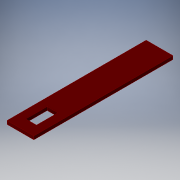
# Autodesk Inventor part: Brazo_Superior
Saved by Autodesk Inventor 2019 (Build 230136000, 136)
## iProperties
Created: 2020-02-09
Part Number: Brazo_Superior
Material: Generic
Document SubType Name: Modeling
Designer: Omar
Density: 1 g/cm^3
Appearance: Default
Author: Omar
Autodesk Inventor part; units mm, degrees
ref_plane "YZ Plane" through (0, 0, 0) normal (1, 0, 0) x (0, 1, 0)
ref_plane "XZ Plane" through (0, 0, 0) normal (0, 1, 0) x (-1, 0, 0)
ref_plane "XY Plane" through (0, 0, 0) normal (0, 0, 1) x (1, 0, 0)
sketch "Sketch1" plane through (0, 0, 0) normal (0, 1, 0) x (-1, 0, 0)
  line L0 (-7.5, -95.91) -> (-7.5, -99.09)
  line L1 (1.59, -90) -> (-1.59, -90)
  line L2 (-1.59, -90) -> (-1.59, -105)
  line L3 (-1.59, -105) -> (1.59, -105)
  line L4 (1.59, -105) -> (1.59, -90)
  line L5 (-1.59, -90) -> (1.59, -105) construction
  line L6 (7.5, -95.91) -> (-7.5, -95.91)
  line L7 (-7.5, -99.09) -> (7.5, -99.09)
  line L8 (7.5, -99.09) -> (7.5, -95.91)
  line L9 (1.59, -90) -> (-1.59, -105) construction
  line L10 (-5, 10) -> (5, 10)
  line L11 (5, 10) -> (5, -10)
  line L12 (5, -10) -> (-5, -10)
  line L13 (-5, -10) -> (-5, 10)
  line L14 (-5, 10) -> (5, -10) construction
  line L15 (5, 10) -> (-5, -10) construction
  line L16 (12.5, 20) -> (-12.5, 20)
  line L17 (-12.5, 20) -> (-12.5, -110)
  line L18 (-12.5, -110) -> (12.5, -110)
  line L19 (12.5, -110) -> (12.5, 20)
  point P0 (0, 0)
  point P1 (0, 0)
  point P2 (0, -97.5)
  point P3 (0, 0)
  dimension "d16" = 15
  dimension "d18" = 3.18
  dimension "d19" = 15
  dimension "d20" = 7.5
  dimension "d21" = 1.59
  dimension "d24" = 10
  dimension "d25" = 20
  dimension "d26" = 25
  dimension "d27" = 130
  dimension "d28" = 20
  dimension "d29" = 12.5
  dimension "d30" = 12.5
  dimension "d31" = 12.5
  dimension "d32" = 3.18
  constraints: 40 end point, 8 parallel, 5 midpoint, 4 horizontal, 4 perpendicular, 1 coincident
  measures "d16" distance of L7.end L0.end
  measures "d18" distance of L3.end L2.end
  measures "d19" distance of L2.end L1.end
  measures "d20" distance from line of L8 point (0, -97.5)
  measures "d21" distance from line of L7 point (0, -97.5)
  measures "d24" distance of L11.end L12.end
  measures "d25" distance of L10.end L11.end
  measures "d26" distance of L18.end L17.end
  measures "d27" distance of L18.end L16.start
  measures "d28" distance from line of L16 point (0, 0)
  measures "d29" distance from line of L19 point (0, 0)
  measures "d30" distance from line of L18 point (0, -97.5)
  measures "d31" distance from line of L17 point (0, -97.5)
  measures "d32" distance of L7.end L6.start
extrude "Extrusion2" add sketch "Sketch1" along normal blind 3.18 contours L6 L2 L7 L0 | L6 L4 L7 L2 | L2 L1 L4 L6 | L7 L4 L3 L2 | L6 L8 L7 L4 | L19 L18 L17 L16
body "Solid2"
